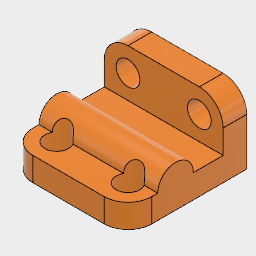
Detailed Drawing Challenge2_ CSA011070∩╗┐ (Autodesk Fusion 360 design; units mm, degrees)
Autodesk Fusion 360 part; units mm, degrees
sketch "Sketch1" plane through (0, 0, 0) normal (1, 0, 0) x (0, 0, -1)
  arc A0 (-19.05, -50.8) -> (19.05, -50.8) centre (0, -50.8) cw
  line L0 (19.05, -50.8) -> (50.8, -50.8)
  line L1 (-50.8, -50.8) -> (-19.05, -50.8)
  line L2 (50.8, -50.8) -> (50.8, 0)
  line L3 (50.8, 0) -> (76.2, 0)
  line L4 (76.2, 0) -> (76.2, -76.2)
  line L5 (76.2, -76.2) -> (-50.8, -76.2)
  line L6 (-50.8, -76.2) -> (-50.8, -50.8)
  point P0 (50.8, 0)
  dimension "d13" = 25.4
  dimension "d14" = 25.4
  measures "d13" distance of L5.end L1.start
  measures "d14" distance of P0 L3.end
extrude "Extrude1" add sketch "Sketch1" along normal mid plane 127
fillet "Fillet1" radius 25.4 4 edges at (-63.5, 0, -63.5) (63.5, 0, -63.5) (-63.5, -63.5, 50.8) (63.5, -63.5, 50.8)
sketch "Sketch2" plane through (0, -76.2, 0) normal (0, -1, 0) x (1, 0, 0)
  arc A0 (63.5, 25.4) -> (38.1, 50.8) centre (38.1, 25.4) ccw
  line L0 (38.1, 50.8) -> (-38.1, 50.8)
  arc A1 (-38.1, 50.8) -> (-63.5, 25.4) centre (-38.1, 25.4) ccw
  line L1 (-63.5, 25.4) -> (-63.5, -76.2)
  line L2 (-63.5, -76.2) -> (63.5, -76.2)
  line L3 (63.5, -76.2) -> (63.5, 25.4)
  circle A2 centre (-38.1, 25.4) radius 12.7
  circle A3 centre (38.1, 25.4) radius 12.7
  dimension "d2" = 25.4
  measures "d2" diameter of A3
extrude "Extrude2" cut sketch "Sketch2" against normal blind 66.04 contours A2 | A3
sketch "Sketch3" plane through (0, 0, -76.2) normal (0, 0, -1) x (-1, 0, 0)
  arc A0 (-38.1, 0) -> (-63.5, -25.4) centre (-38.1, -25.4) ccw
  line L0 (-63.5, -25.4) -> (-63.5, -76.2)
  line L1 (-63.5, -76.2) -> (63.5, -76.2)
  line L2 (63.5, -76.2) -> (63.5, -25.4)
  arc A1 (63.5, -25.4) -> (38.1, 0) centre (38.1, -25.4) ccw
  line L3 (38.1, 0) -> (-38.1, 0)
  circle A2 centre (-38.1, -25.4) radius 12.7
  circle A3 centre (38.1, -25.4) radius 12.7
  dimension "d5" = 25.4
  measures "d5" diameter of A3
extrude "Extrude3" cut sketch "Sketch3" against normal blind 30.48 contours A2 | A3
